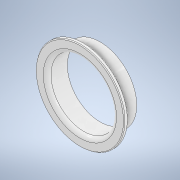
# Autodesk Inventor part: Buje de base soporte
Saved by Autodesk Inventor 2021 (Build 250183000, 183)
## iProperties
Created: 2021-04-15
Part Number: Buje de base soporte
Material: Genérico
Document SubType Name: Modeling
Designer: Leonardo Fabio Mercado Benítez
Density: 1 g/cm^3
Appearance: Valor por defecto
Author: Leonardo Fabio Mercado Benítez
Autodesk Inventor part; units mm, degrees
ref_plane "YZ Plane" through (0, 0, 0) normal (1, 0, 0) x (0, 1, 0)
ref_plane "XZ Plane" through (0, 0, 0) normal (0, 1, 0) x (-1, 0, 0)
ref_plane "XY Plane" through (0, 0, 0) normal (0, 0, 1) x (1, 0, 0)
sketch "Boceto1" plane through (0, 0, 0) normal (0, 0, 1) x (1, 0, 0)
  circle A0 centre (0, 0) radius 12.7
  circle A1 centre (0, 0) radius 14.2
  dimension "d0" = 25.4
  dimension "d1" = 28.4
  constraints: 2 centre point, 2 coincident
  measures "d0" diameter of A0
  measures "d1" diameter of A1
extrude "Extrusión1" add sketch "Boceto1" along normal mid plane 6.35
sketch "Boceto2" plane through (0, 0, 0) normal (1, 0, 0) x (0, 1, 0)
  line L0 (14.2, 3.175) -> (16.9, 3.175)
  line L1 (17.2, 3.475) -> (17.2, 4.375)
  line L2 (16.9, 4.675) -> (14.2, 4.675)
  arc A0 (14.2, 4.675) -> (12.7, 3.175) centre (14.2, 3.175) ccw
  arc A1 (16.9, 3.175) -> (17.2, 3.475) centre (16.9, 3.475) ccw
  arc A2 (17.2, 4.375) -> (16.9, 4.675) centre (16.9, 4.375) ccw
  line L3 (14.2, 3.175) -> (12.7, 3.175)
  line L4 (0, -0.9971) -> (0, 5.9828) projected
  point P0 (0, 0)
  point P1 (17.2, 3.175)
  point P2 (17.2, 4.675)
  dimension "d4" = 3
  dimension "d5" = 1.5
  dimension "d6" = 3
  dimension "d7" = 0.3
  constraints: 8 end point, 6 point on circle, 4 point on line, 4 tangent, 3 centre point, 1 coincident, 1 equal radius, 1 horizontal, 1 perpendicular, 1 vertical
  measures "d4" distance of L0.start point (17.2, 3.175)
  measures "d5" distance of point (17.2, 3.175) point (17.2, 4.675)
  measures "d6" distance of point (17.2, 4.675) L2.end
  measures "d7" radius of A1
revolve "Revolución1" add sketch "Boceto2" angle 360 about axis through (0, 0, -10) along (0, 0, 1)
